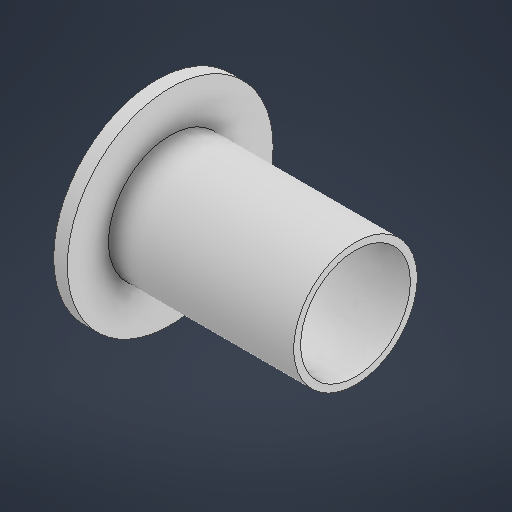
# Autodesk Inventor part: Spulenhalter-Ph-L
Saved by Autodesk Inventor 2026.1 (Build 301233000, 233)
## iProperties
Created: 2025-12-08
Part Number: Spulenhalter-Ph-L
Material: Generisch
Document SubType Name: Modeling
Designer: rebsa
Density: 1 g/cm^3
Appearance: Vorgabe
Author: rebsa
Autodesk Inventor part; units mm, degrees
ref_plane "YZ Plane" through (0, 0, 0) normal (1, 0, 0) x (0, 1, 0)
ref_plane "XZ Plane" through (0, 0, 0) normal (0, 1, 0) x (-1, 0, 0)
ref_plane "XY Plane" through (0, 0, 0) normal (0, 0, 1) x (1, 0, 0)
sketch "Skizze1" plane through (0, 0, 0) normal (1, 0, 0) x (0, 1, 0)
  circle A0 centre (0, 0) radius 8
  line L0 (-12.6, 0) -> (12.6, 0) projected
  line L1 (0, -12.6) -> (0, 12.6) projected
  circle A1 centre (0, 0) radius 9
  dimension "d0" = 16
  dimension "d1" = 18
  constraints: 2 centre point, 1 coincident, 1 concentric
  measures "d0" diameter of A0
  measures "d1" diameter of A1
extrude "Extrusion1" add sketch "Skizze1" along normal blind 27 contours L0 A1 L1 A0 | A0 L1 A1 L0 | A0 L0 A1 L1 | L1 A1 L0 A0
sketch "Skizze3" plane through (0, 0, 0) normal (-1, 0, 0) x (0, 0, 1)
  circle A0 centre (0, 0) radius 8
  circle A1 centre (0, 0) radius 15
  circle A2 centre (0, 0) radius 8 projected
  dimension "d7" = 30
  constraints: 3 concentric, 2 centre point
  measures "d7" diameter of A1
extrude "Extrusion3" add sketch "Skizze3" along normal blind 2
